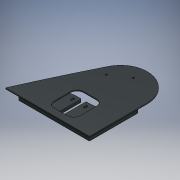
# Autodesk Inventor part: D0001
Saved by Autodesk Inventor 2017 (Build 210142000, 142)
## iProperties
Part Number: D0001
Material: SS41
Document SubType Name: Modeling
Designer: G
Density: 7.85 g/cm^3
Appearance: 鐵灰色
Author: G
Autodesk Inventor part; units mm, degrees
ref_plane "YZ Plane" through (0, 0, 0) normal (1, 0, 0) x (0, 1, 0)
ref_plane "XZ Plane" through (0, 0, 0) normal (0, 1, 0) x (-1, 0, 0)
ref_plane "XY Plane" through (0, 0, 0) normal (0, 0, 1) x (1, 0, 0)
sketch "草圖1" plane through (0, 0, 0) normal (0, 0, 1) x (1, 0, 0)
  arc A0 (0, 45) -> (-45, 0) centre (0, 0) ccw
  arc A1 (0, 65) -> (-65, 0) centre (0, 0) ccw
  line L0 (0, 65) -> (0, 0)
  line L1 (0, 0) -> (-65, 0)
  arc A2 (18, 45) -> (60.0968, 74.0984) centre (18, 90) ccw
  line L2 (0, 0) -> (63, 0)
  line L3 (63, 73.5683) -> (63, 0)
  arc A3 (63, 73.5683) -> (60.0968, 74.0984) centre (61.5, 73.5683) ccw
  line L4 (13, 45) -> (13, 10)
  line L5 (13, 10) -> (5, 10)
  line L6 (5, 10) -> (5, 45)
  line L7 (0, 45) -> (5, 45)
  line L8 (13, 45) -> (18, 45)
  dimension "d0" = 20
  dimension "d7" = 1.5
  dimension "d11" = 10
  dimension "d12" = 8
  dimension "d15" = 5
  dimension "d16" = 5
  dimension "d17" = 35
  dimension "d24" = 45
  constraints: 18 end point, 8 point on circle, 5 tangent, 4 centre point, 3 horizontal, 3 vertical, 2 coincident, 2 point on line, 1 parallel, 1 perpendicular
  measures "d0" radial gap between concentric circles of A0 A1
  measures "d7" radius of A3
  measures "d11" distance between parallel lines of L2 L5
  measures "d12" distance between parallel lines of L6 L4
  measures "d15" distance from line of L6 L7.start
  measures "d16" distance of L4.start L8.end
  measures "d17" distance of L4.start L4.end
  measures "d24" radius of A2
extrude "擠出1" add sketch "草圖1" along normal mid plane 5 contours L0 L1 A0 | L7 L6 L5 L4 L8 A2 A3 L3 L2 L0
sketch "草圖3" plane through (0, 0, 2.5) normal (0, 0, 1) x (1, 0, 0)
  line L0 (-1.6, 39.7) -> (-0.5, 39.7) construction
  arc A0 (-0.5, 36.5) -> (-0.5, 39.7) centre (-0.5, 38.1) ccw construction
  line L1 (18.5, 39.7) -> (19.6, 39.7) construction
  line L2 (-1.05, 39.6) -> (-1.05, 36.6) construction
  line L3 (-2.65, 39.6) -> (-2.65, 36.6)
  line L4 (0.55, 36.6) -> (0.55, 39.6)
  arc A1 (0.55, 39.6) -> (-2.65, 39.6) centre (-1.05, 39.6) ccw
  arc A2 (-2.65, 36.6) -> (0.55, 36.6) centre (-1.05, 36.6) ccw
  line L5 (19.05, 39.6) -> (19.05, 36.6) construction
  line L6 (17.45, 39.6) -> (17.45, 36.6)
  line L7 (20.65, 36.6) -> (20.65, 39.6)
  arc A3 (20.65, 39.6) -> (17.45, 39.6) centre (19.05, 39.6) ccw
  arc A4 (17.45, 36.6) -> (20.65, 36.6) centre (19.05, 36.6) ccw
  point P0 (0, 0)
  point P1 (-1.05, 38.1)
  point P2 (19.05, 38.1)
  point P3 (-1.05, 39.7)
  point P4 (19.05, 39.7)
  dimension "d18" = 3.2
  dimension "d19" = 3.2
  dimension "d20" = 3
  dimension "d21" = 3
  constraints: 16 end point, 8 point on circle, 8 tangent, 4 centre point, 4 midpoint, 3 parallel, 2 horizontal alignment, 2 vertical alignment, 1 perpendicular
  measures "d18" distance between parallel lines of L4 L3
  measures "d19" distance between parallel lines of L7 L6
  measures "d20" distance of L3.start L3.end
  measures "d21" distance of L6.start L6.end
extrude "擠出3" cut sketch "草圖3" along normal through all both and the other way through all
sketch "草圖4" plane through (0, 0, 0) normal (0, 0, 1) x (1, 0, 0)
  circle A0 centre (152.9499, 110.8116) radius 22.5
  arc A1 (18, 45) -> (60.0968, 74.0984) centre (18, 90) ccw construction
  arc A2 (0, 45) -> (-45, 0) centre (0, 0) ccw construction
  arc A3 (-17, 80.687) -> (39.435, 120) centre (-36.3223, 168.5884) ccw
  line L0 (63, 73.5683) -> (63, 0) construction
  line L1 (63, 73.5683) -> (63, 177.2446) construction
  arc A4 (63, 119.0046) -> (27.9571, 105.595) centre (60.0968, 74.0984) ccw construction
  arc A5 (-17, 101.308) -> (14.0679, 120) centre (-36.3223, 168.5884) ccw construction
  line L2 (14.0679, 120) -> (39.435, 120) construction
  line L3 (-17, 101.308) -> (-17, 80.687) construction
  arc A6 (-0.1074, 86.1961) -> (-26.2057, 36.5823) centre (18, 45) ccw construction
  line L4 (63, 0) -> (-45, 0) projected
  arc A7 (-17, 90.9569) -> (27.2322, 120) centre (-36.3223, 168.5884) ccw construction
  circle A8 centre (-5.7306, 94.6685) radius 1.6
  circle A9 centre (19.3468, 111.1345) radius 1.6
  line L5 (-5.7306, 94.6685) -> (19.3468, 111.1345) construction
  line L6 (6.8081, 102.9015) -> (7.5869, 101.7155) construction
  arc A10 (39.435, 120) -> (-17, 80.687) centre (17.728, 90.9975) ccw
  dimension "d25" = 45
  dimension "d28" = 45
  dimension "d29" = 90
  dimension "d30" = 20
  dimension "d32" = 120
  dimension "d33" = 80
  dimension "d34" = 10
  dimension "d35" = 30
  dimension "d36" = 3.2
  constraints: 20 point on circle, 10 end point, 9 centre point, 3 equal radius, 3 point on line, 2 coincident, 2 tangent, 2 vertical, 1 horizontal, 1 midpoint, 1 perpendicular, 1 other
  measures "d25" diameter of A0
  measures "d28" radius of A4
  measures "d29" radius of A3
  measures "d30" radial gap between concentric circles of A3 A5
  measures "d32" distance between parallel lines of L4 L2
  measures "d33" distance between parallel lines of L0 L3
  measures "d34" radial gap between concentric circles of A3 A7
  measures "d35" distance of L5.end L5.start
  measures "d36" diameter of A8
extrude "擠出4" add sketch "草圖4" against normal up to surface (5 mm away) from surface at 2.5 separate body contours A10 A3
sketch "草圖5" plane through (0, 0, 2.5) normal (0, 0, 1) x (1, 0, 0)
  arc A0 (18, 45) -> (60.0968, 74.0984) centre (18, 90) ccw construction
  line L0 (18, 45) -> (13, 45) construction
  line L1 (5, 45) -> (0, 45) construction
  arc A1 (0, 45) -> (-45, 0) centre (0, 0) ccw construction
  line L2 (5, 45) -> (13, 45) construction
  line L3 (-65, 0) -> (63, 0)
  line L4 (63, 88.8671) -> (63, 0)
  line L5 (-1, 55) -> (19, 55)
  line L6 (29, 45) -> (29, 20)
  line L7 (19, 10) -> (-1, 10)
  line L8 (-11, 20) -> (-11, 45)
  line L9 (13, 10) -> (5, 10) construction
  arc A2 (-1, 55) -> (-11, 45) centre (-1, 45) ccw
  arc A3 (29, 45) -> (19, 55) centre (19, 45) ccw
  arc A4 (19, 10) -> (29, 20) centre (19, 20) ccw
  arc A5 (-11, 20) -> (-1, 10) centre (-1, 20) ccw
  arc A6 (63, 88.8671) -> (-14.6906, 107.1646) centre (22, 88.8671) ccw
  arc A7 (-14.6906, 107.1646) -> (-65, 0) centre (2221.6229, -1008.0847) ccw
  circle A8 centre (-5.7306, 94.6685) radius 1.6 projected
  circle A9 centre (19.3468, 111.1345) radius 1.6 projected
  arc A10 (39.435, 120) -> (-17, 80.687) centre (17.728, 90.9975) ccw construction
  point P0 (-11, 55)
  point P1 (29, 55)
  point P2 (9, 10)
  point P3 (-21.8569, 69.1091)
  dimension "d41" = 40
  dimension "d42" = 10
  dimension "d45" = 10
  dimension "d47" = 20
  dimension "d48" = 41
  constraints: 14 end point, 13 point on circle, 12 tangent, 6 centre point, 5 point on line, 3 equal radius, 3 horizontal, 2 midpoint, 2 parallel, 2 perpendicular, 1 coincident
  measures "d41" distance of point (-11, 55) point (29, 55)
  measures "d42" radius of A2
  measures "d45" distance between parallel lines of L2 L5
  measures "d47" distance of A1.end L3.start
  measures "d48" radius of A6
extrude "擠出5" add sketch "草圖5" along normal blind 2 separate body
